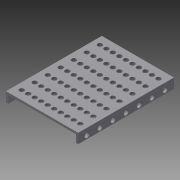
# Autodesk Inventor part: RPiCaseTopV2
Saved by Autodesk Inventor 2015 (Build 190159000, 159)
## iProperties
Created: 2016-02-20
Part Number: RPiCaseTopV2
Material: Generic
Document SubType Name: Modeling
Designer: Hatch
Density: 1 g/cm^3
Appearance: Default
Author: Hatch
Autodesk Inventor part; units mm, degrees
ref_plane "YZ Plane" through (0, 0, 0) normal (1, 0, 0) x (0, 1, 0)
ref_plane "XZ Plane" through (0, 0, 0) normal (0, 1, 0) x (-1, 0, 0)
ref_plane "XY Plane" through (0, 0, 0) normal (0, 0, 1) x (1, 0, 0)
sketch "Sketch1" plane through (0, 0, 0) normal (0, 1, 0) x (-1, 0, 0)
  line L0 (0, 0) -> (62.25, 0)
  line L1 (62.25, 0) -> (62.25, -88.25)
  line L2 (62.25, -88.25) -> (0, -88.25)
  line L3 (0, -88.25) -> (0, 0)
  dimension "d0" = 62.25
  dimension "d1" = 88.25
  constraints: 8 end point, 2 parallel, 1 horizontal, 1 perpendicular
  measures "d0" distance of L1.end L2.end
  measures "d1" distance of L0.end L1.end
extrude "Extrusion1" add sketch "Sketch1" along normal blind 2
sketch "Sketch2" plane through (0, 2, 0) normal (0, 1, 0) x (1, 0, 0)
  line L0 (-62.25, 0) -> (-62.0625, 0)
  line L1 (-62.25, 0) -> (0, 0) projected
  line L2 (0, 88.25) -> (-62.25, 88.25) projected
  circle A0 centre (-59.0445, 2.125) radius 2.125
  dimension "d4" = 0.1875
  dimension "d7" = 4.25
  constraints: 2 end point, 1 centre point, 1 point on line
  measures "d4" distance of L0.start L0.end
  measures "d7" diameter of A0
extrude "Extrusion2" cut sketch "Sketch2" against normal blind 2
pattern_linear "Rectangular Pattern1" count 15 spacing 6 along (0, 0, -1) count 10 spacing 6 along (1, 0, 0) of "Extrusion2"
sketch "Sketch3" plane through (-62.25, 0, -88.25) normal (-1, 0, 0) x (0, 0, 1)
  line L0 (88.25, 0) -> (0, 0)
  line L1 (0, 0) -> (0, 2)
  line L2 (0, 2) -> (88.25, 2)
  line L3 (88.25, 2) -> (88.25, 0)
  constraints: 8 end point, 2 parallel, 1 horizontal, 1 perpendicular
extrude "Extrusion3" add sketch "Sketch3" along normal blind 3.1
sketch "Sketch4" plane through (0, 0, 0) normal (1, 0, 0) x (0, 0, -1)
  line L0 (0, 2) -> (88.25, 2)
  line L1 (88.25, 2) -> (88.25, 0)
  line L2 (88.25, 0) -> (0, 0)
  line L3 (0, 0) -> (0, 2)
  constraints: 8 end point, 2 parallel, 1 horizontal, 1 perpendicular
extrude "Extrusion4" add sketch "Sketch4" along normal blind 1.1
sketch "Sketch5" plane through (0, 0, 0) normal (0, -1, 0) x (1, 0, 0)
  line L0 (-5.0445, -88.25) -> (1.1, -88.25) projected
  line L1 (1.1, 0) -> (-0.9, 0)
  line L2 (-0.9, 0) -> (-0.9, -88.25)
  line L3 (-0.9, -88.25) -> (1.1, -88.25)
  line L4 (1.1, -88.25) -> (1.1, 0)
  point P0 (0, 0)
  dimension "d20" = 2
  constraints: 8 end point, 2 parallel, 1 horizontal, 1 perpendicular, 1 point on line
  measures "d20" distance of L3.end L2.end
extrude "Extrusion5" add sketch "Sketch5" along normal blind 7
sketch "Sketch6" plane through (0, 0, 0) normal (0, -1, 0) x (1, 0, 0)
  line L0 (-59.0445, 0) -> (-65.35, 0) projected
  line L1 (-65.35, -88.25) -> (-63.35, -88.25)
  line L2 (-63.35, -88.25) -> (-63.35, 0)
  line L3 (-63.35, 0) -> (-65.35, 0)
  line L4 (-65.35, 0) -> (-65.35, -88.25)
  point P0 (0, 0)
  dimension "d23" = 2
  constraints: 8 end point, 2 parallel, 1 horizontal, 1 perpendicular, 1 point on line
  measures "d23" distance of L3.end L2.end
extrude "Extrusion6" add sketch "Sketch6" along normal blind 7
sketch "Sketch7" plane through (-65.35, 0, -88.25) normal (-1, 0, 0) x (0, 0, 1)
  line L0 (88.25, -7) -> (0, -7) projected
  line L1 (59.4144, -7) -> (59.4144, -6.125)
  line L2 (88.25, 2) -> (0, 2) projected
  line L3 (59.4144, -6.125) -> (59.4144, -4)
  line L4 (88.25, -7) -> (86.125, -7)
  line L5 (0, -7) -> (88.25, -7) projected
  circle A0 centre (86.125, -4) radius 2.125
  point P0 (88.25, 0)
  dimension "d26" = 0.875
  dimension "d27" = 2.125
  dimension "d28" = 2.125
  dimension "d29" = 4.25
  constraints: 6 end point, 3 point on line, 1 centre point, 1 perpendicular
  measures "d26" distance of L1.start L1.end
  measures "d27" distance of L1.end L3.end
  measures "d28" distance of L0.start L4.end
  measures "d29" diameter of A0
extrude "Extrusion7" cut sketch "Sketch7" against normal through all
pattern_linear "Rectangular Pattern2" count 15 spacing 6 along (0, 0, -1) of "Extrusion7"
sketch "Sketch8" plane through (0, 2, 0) normal (0, 1, 0) x (1, 0, 0)
  circle A0 centre (-59.0445, 2.125) radius 2.125 projected
  circle A1 centre (-59.0445, -9.875) radius 2.125
  circle A2 centre (-59.0445, -9.875) radius 2.125
  point P0 (0, 0)
  point P1 (-59.0445, 0)
  dimension "d36" = 4.25
  constraints: 2 centre point, 1 coincident, 1 concentric, 1 vertical alignment
  measures "d36" diameter of A1
extrude "Extrusion8" add sketch "Sketch8" against normal blind 2 contours A1
pattern_linear "Rectangular Pattern3" count 9 spacing 12 along (0, 0, -1) count 10 spacing 6 along (1, 0, 0) of "Extrusion8"
sketch "Sketch9" plane through (0, 2, 0) normal (0, 1, 0) x (1, 0, 0)
  line L0 (-62.5545, -15.6579) -> (0, -15.6579)
  line L1 (0, -15.6579) -> (0, -4.9567)
  line L2 (0, -4.9567) -> (-62.5545, -4.9567)
  line L3 (-62.5545, -4.9567) -> (-62.5545, -15.6579)
  point P0 (0, 0)
  constraints: 8 end point, 2 parallel, 1 horizontal, 1 perpendicular
extrude "Extrusion9" cut sketch "Sketch9" against normal blind 2
sketch "Sketch10" plane through (1.1, 2, 0) normal (1, 0, 0) x (0, 0, -1)
  circle A0 centre (2.125, -6) radius 2.125 projected
  circle A1 centre (-9.875, -6) radius 2.125
  circle A2 centre (-9.875, -6) radius 2.125
  point P0 (0, -2)
  point P1 (0, -6)
  dimension "d48" = 4.25
  constraints: 2 centre point, 1 coincident, 1 concentric, 1 horizontal alignment
  measures "d48" diameter of A1
extrude "Extrusion10" add sketch "Sketch10" against normal blind 2 contours A1
pattern_linear "Rectangular Pattern4" count 9 spacing 12 along (0, 0, -1) of "Extrusion10"
sketch "Sketch11" plane through (-65.35, 2, -88.25) normal (-1, 0, 0) x (0, 0, 1)
  circle A0 centre (86.125, -6) radius 2.125 projected
  circle A1 centre (98.125, -6) radius 2.125
  circle A2 centre (98.125, -6) radius 2.125
  point P0 (88.25, -2)
  point P1 (88.25, -6)
  dimension "d55" = 4.25
  constraints: 2 centre point, 1 coincident, 1 concentric, 1 horizontal alignment
  measures "d55" diameter of A1
extrude "Extrusion11" add sketch "Sketch11" against normal blind 2 contours A1
pattern_linear "Rectangular Pattern5" count 9 spacing 12 along (0, 0, -1) of "Extrusion11"
sketch "Sketch12" plane through (1.1, 0, 0) normal (1, 0, 0) x (0, 0, -1)
  line L0 (-12.8358, -10.1364) -> (-4.0215, -10.1364)
  line L1 (-4.0215, -10.1364) -> (-4.0215, 1.7629)
  line L2 (-4.0215, 1.7629) -> (-12.8358, 1.7629)
  line L3 (-12.8358, 1.7629) -> (-12.8358, -10.1364)
  point P0 (0, 0)
  constraints: 8 end point, 2 parallel, 1 horizontal, 1 perpendicular
extrude "Extrusion12" cut sketch "Sketch12" against normal through all
body "Solid1"
